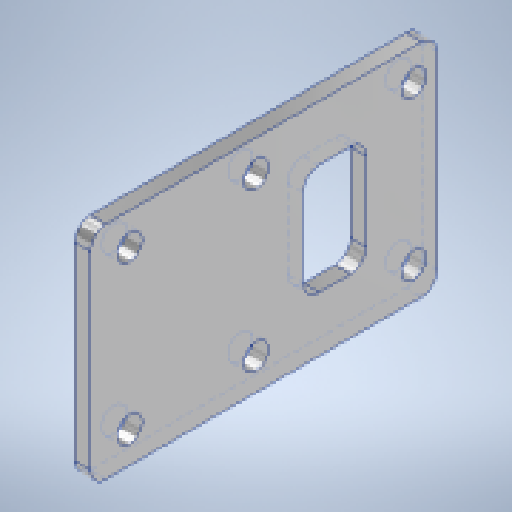
# Autodesk Inventor part: 2mm_connect
Saved by Autodesk Inventor 2025 (Build 290162000, 162)
## iProperties
Created: 2025-02-24
Part Number: 2mm_connect
Material: アルミニウム 6061
Document SubType Name: Modeling
Designer: Zhopa
Density: 2.7 g/cm^3
Appearance: アルミニウム - フラット
Mass: 5.78742 g
Surface Area: 26.2639 cm^2
Volume: 2.14349 cm^3
Author: Zhopa
Autodesk Inventor part; units mm, degrees
ref_plane "YZ Plane" through (0, 0, 0) normal (1, 0, 0) x (0, 1, 0)
ref_plane "XZ Plane" through (0, 0, 0) normal (0, 1, 0) x (-1, 0, 0)
ref_plane "XY Plane" through (0, 0, 0) normal (0, 0, 1) x (1, 0, 0)
sketch "Sketch1" plane through (0, 0, 0) normal (1, 0, 0) x (0, 1, 0)
  line L0 (-14, 22) -> (14, 22)
  line L1 (14, 22) -> (14, -22)
  line L2 (14, -22) -> (-14, -22)
  line L3 (-14, -22) -> (-14, 22)
  line L4 (-14, 22) -> (14, -22) construction
  line L5 (14, 22) -> (-14, -22) construction
  circle A0 centre (10, 17) radius 1.6
  circle A1 centre (-10, 17) radius 1.6
  circle A2 centre (-10, 1) radius 1.6
  circle A3 centre (10, 1) radius 1.6
  circle A4 centre (10, -19) radius 1.6
  circle A5 centre (-10, -19) radius 1.6
  line L6 (-7, -13) -> (7, -13)
  line L7 (7, -13) -> (7, -5)
  line L8 (7, -5) -> (-7, -5)
  line L9 (-7, -5) -> (-7, -13)
  line L10 (-7, -13) -> (7, -5) construction
  line L11 (7, -13) -> (-7, -5) construction
  point P0 (0, 0)
  point P1 (10, -6)
  point P2 (-10, 24)
  point P3 (0, -9)
  dimension "d0" = 28
  dimension "d1" = 44
  dimension "d2" = 4
  dimension "d3" = 3
  dimension "d4" = 4
  dimension "d5" = 20
  dimension "d6" = 5
  dimension "d7" = 3.2
  dimension "d8" = 3.2
  dimension "d9" = 3.2
  dimension "d10" = 3.2
  dimension "d11" = 3.2
  dimension "d12" = 3.2
  dimension "d16" = 10
  dimension "d17" = 10
  dimension "d18" = 14
  dimension "d19" = 8
  dimension "d20" = 0
  dimension "d21" = 0
  dimension "d22" = 0
  dimension "d23" = 20
  dimension "d24" = 5
  dimension "d25" = 3
  constraints: 24 end point, 6 centre point, 4 midpoint, 4 parallel, 2 horizontal, 2 perpendicular, 1 coincident
  measures "d0" distance of L1.end L2.end
  measures "d1" distance of L0.end L1.end
  measures "d2" distance from line of L1 point (10, -19)
  measures "d3" distance from line of L2 point (10, -19)
  measures "d4" distance from line of L3 point (-10, -19)
  measures "d5" distance of point (-10, -19) point (-10, 1)
  measures "d6" distance from line of L0 point (10, 17)
  measures "d7" diameter of A0
  measures "d8" diameter of A1
  measures "d9" diameter of A2
  measures "d10" diameter of A3
  measures "d11" diameter of A4
  measures "d12" diameter of A5
  measures "d16" horizontal distance of point (0, -9) point (10, -19)
  measures "d17" horizontal distance of point (0, -9) point (10, -19)
  measures "d18" distance of L8.end L7.end
  measures "d19" distance of L7.end L6.end
  measures "d20" distance of point (10, -19) A4.centre
  measures "d21" distance of point (-10, -19) A5.centre
  measures "d22" distance of point (-10, 1) A2.centre
  measures "d23" distance of A4.centre A3.centre
  measures "d24" distance from line of L0 A1.centre
  measures "d25" distance from line of L2 A5.centre
extrude "Extrusion1" add sketch "Sketch1" along normal blind 2
fillet "Fillet1" radius 2 8 edges at (1, 14, 22) (1, 14, -22) (1, -14, -22) (1, -14, 22) (1, 7, -5) (1, 7, -13) (1, -7, -5) (1, -7, -13)
equation "\"d23\" = d5"
equation "\"d24\" = d6"
body "Solid1"
